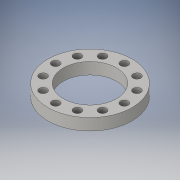
# Autodesk Inventor part: vexSupportRing
Saved by Autodesk Inventor 2016 SP1 (Build 200210100, 210)
## iProperties
Created: 2015-11-19
Part Number: vexSupportRing
Material: Generic
Document SubType Name: Modeling
Designer: steele
Density: 1 g/cm^3
Appearance: Default
Author: steele
Autodesk Inventor part; units mm, degrees
ref_plane "YZ Plane" through (0, 0, 0) normal (1, 0, 0) x (0, 1, 0)
ref_plane "XZ Plane" through (0, 0, 0) normal (0, 1, 0) x (-1, 0, 0)
ref_plane "XY Plane" through (0, 0, 0) normal (0, 0, 1) x (1, 0, 0)
sketch "Sketch1" plane through (0, 0, 0) normal (0, 1, 0) x (-1, 0, 0)
  circle A0 centre (0, 0) radius 51.5874
  circle A1 centre (0, 0) radius 81.2419
  dimension "d0" = 103.1748
  dimension "d1" = 162.4838
  constraints: 2 centre point, 2 coincident
  measures "d0" diameter of A0
  measures "d1" diameter of A1
extrude "Extrusion1" add sketch "Sketch1" along normal blind 22.479
sketch "Sketch2" plane through (0, 22.479, 0) normal (0, 1, 0) x (1, 0, 0)
  circle A0 centre (66.4146, 0) radius 7.4136
  circle A1 centre (57.5168, 33.2073) radius 7.4136
  circle A2 centre (33.2073, 57.5168) radius 7.4136
  circle A3 centre (0, 66.4146) radius 7.4136
  circle A4 centre (-33.2073, 57.5168) radius 7.4136
  circle A5 centre (-57.5168, 33.2073) radius 7.4136
  circle A6 centre (-66.4146, 0) radius 7.4136
  circle A7 centre (-57.5168, -33.2073) radius 7.4136
  circle A8 centre (-33.2073, -57.5168) radius 7.4136
  circle A9 centre (0, -66.4146) radius 7.4136
  circle A10 centre (33.2073, -57.5168) radius 7.4136
  circle A11 centre (57.5168, -33.2073) radius 7.4136
  point P0 (0, 0)
  dimension "d4" = 14.8272
  dimension "d6" = 66.4146
  dimension "d9" = 360
  constraints: 12 centre point, 25 other
  measures "d4" diameter of A0
  measures "d6" distance of point (0, 0) A0.centre
extrude "Extrusion2" cut sketch "Sketch2" against normal through all
equation "\"d0\" = insideDiam"
equation "\"d1\" = outsideDiam"
equation "\"d2\" = thickness"
equation "\"d4\" = stregthenHoleDiam"
equation "\"d6\" = shellRadius"
equation "\"d11\" = thickness"
equation "\"thickness\" = 22.479"
equation "\"printerError\" = 0.508"
equation "\"shellWidth\" = -0.5 * insideDiam + 0.5 * outsideDiam"
equation "\"stregthenHoleDiam\" = 0.5 * shellWidth"
equation "\"shellRadius\" = 0.5 * outsideDiam - 0.5 * shellWidth"
equation "\"numberOfHoles\" = 30.48"
equation "\"insideDiam\" = 103.1748"
equation "\"outsideDiam\" = 162.4838"
body "Solid1"
